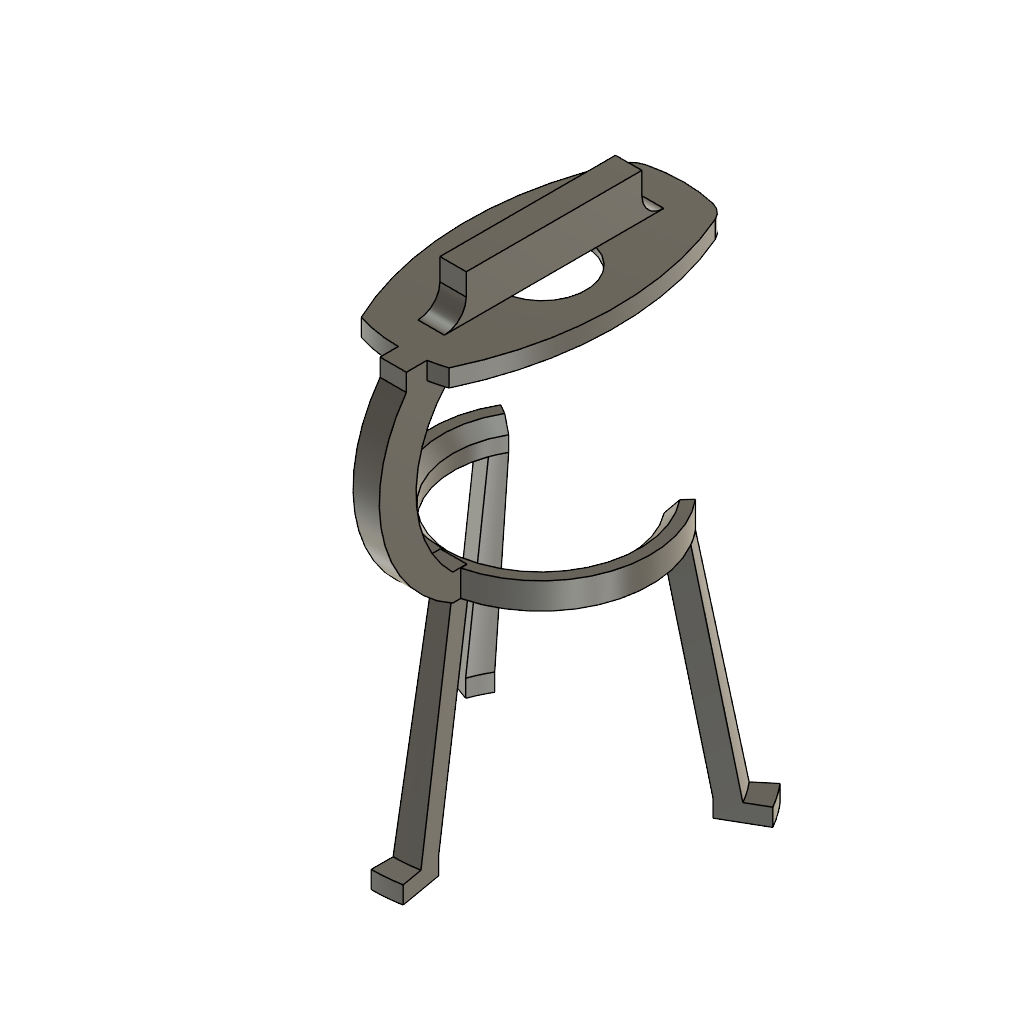
exercise 3 (Autodesk Fusion 360 design; units mm, degrees)
part number: 2026-07-30-11-30-15-373
Autodesk Fusion 360 part; units mm, degrees
note: some values were not read from the file. Set by a fixed rule: which sketch regions a step uses.
sketch "Sketch1" plane through (0, 0, 0) normal (0, 0, 1) x (1, 0, 0)
  circle A0 centre (0, 0) radius 31.75
  circle A1 centre (0, 0) radius 25.4
  dimension "d1" = 63.5
  dimension "d2" = 50.8
  constraint coincident A0.centre A1.centre
  constraint concentric A0 A1
  measures "d1" diameter of A0
  measures "d2" diameter of A1
extrude "Extrude1" add sketch "Sketch1" along normal blind 7.62 makes body 1
chamfer "Chamfer1" distance 3.175 distance2 3.175 1 edges at (-23.6811, 9.185, 7.62) measured on face at (29.4206, -2.8393, 7.62) on bodies 1
sketch "Sketch2" plane through (0, 0, 0) normal (1, 0, 0) x (0, 1, 0)
  arc A0 (-31.115, 59.4476) -> (-33.147, 7.7483) centre (-9.0465, 32.6906) ccw
  arc A1 (-46.5417, 59.4476) -> (-33.147, 0) centre (-13.9818, 35.5511) ccw
  line L0 (-33.147, 7.7483) -> (-33.147, 0)
  line L1 (-33.147, 7.7483) -> (-29.083, 7.7483)
  line L2 (-29.083, 7.7483) -> (-29.083, 0)
  line L3 (-29.083, 0) -> (-33.147, 0)
  line L4 (-33.147, 0) -> (-33.147, 7.7483)
  line L5 (-31.115, 0) -> (-31.115, 59.4476) construction
  line L6 (-46.5417, 59.4476) -> (-31.115, 59.4476)
  constraint tangent A0 A1
  constraint horizontal L1
  constraint vertical L2
  constraint horizontal L3
  constraint vertical L4
  constraint midpoint L3 L5.start
  constraint perpendicular L5 L6
extrude "Extrude2" add sketch "Sketch2" along normal blind 7.62 bodies 1
sketch "Sketch5" plane through (0, 0, 59.4476) normal (0, 0, 1) x (-1, 0, 0)
  line L0 (0, 31.115) -> (0, 46.5417)
  line L1 (0, 46.5417) -> (-7.62, 46.5417)
  line L2 (-7.62, 46.5417) -> (-7.62, 31.115)
  line L3 (-7.62, 31.115) -> (0, 31.115)
  line L4 (12.7, 39.2684) -> (-12.7, 39.2684) construction
  line L5 (-12.7, 39.2684) -> (-12.7, -39.2684) construction
  line L6 (-12.7, -39.2684) -> (12.7, -39.2684) construction
  line L7 (12.7, -39.2684) -> (12.7, 39.2684) construction
  line L8 (12.7, 39.2684) -> (-12.7, -39.2684) construction
  line L9 (-12.7, 39.2684) -> (12.7, -39.2684) construction
  arc A0 (12.7, -39.2684) -> (12.7, 39.2684) centre (-69.8788, 0) ccw
  arc A1 (12.7, 39.2684) -> (-12.7, 39.2684) centre (0, -0.0042) ccw
  arc A2 (-12.7, 39.2684) -> (-12.7, -39.2684) centre (69.8788, 0) ccw
  arc A3 (-12.7, -39.2684) -> (12.7, -39.2684) centre (0, 0.0042) ccw
  line L10 (0, 46.5417) -> (-7.62, 46.5417)
  line L11 (-7.62, 46.5417) -> (-7.62, 31.115)
  line L12 (-7.62, 31.115) -> (0, 31.115)
  line L13 (0, 31.115) -> (0, 46.5417)
  dimension "d20" = 25.4
  dimension "d21" = 78.5368
  dimension "d22" = 91.44
  dimension "d23" = 41.275
  dimension "d24" = 91.44
  dimension "d25" = 41.275
  constraint horizontal L4
  constraint perpendicular L4 L5
  constraint parallel L4 L6
  constraint parallel L5 L7
  constraint coincident L8 origin
  constraint coincident L9 origin
  constraint horizontal L10
  constraint vertical L11
  constraint horizontal L12
  constraint vertical L13
  constraint coincident L2.end L3.start
  constraint coincident L0.end L1.start
  measures "d20" distance of L5.end L6.end
  measures "d21" distance of L4.end L5.end
  measures "d22" radius of A0
  measures "d23" radius of A1
  measures "d24" radius of A2
  measures "d25" radius of A3
extrude "Extrude3" add sketch "Sketch5" along normal blind 5.08 separate body contours L0 L2 L3 A0 A1 A2 A3 L11 L12 L13 makes body 2
extrude "Extrude4" add 1 faces at (2.54, -36.2572, 59.4476) along direction (0, 0, 1) blind 5.08 on bodies 1 bodies 1 2
fillet "Fillet1" radius 6.35 1 edges at (12.7, 39.2684, 61.9876) on bodies 1
fillet "Fillet2" radius 6.35 1 edges at (-12.7, 39.2684, 61.9876) on bodies 1
sketch "Sketch6" plane through (0, 0, 64.5276) normal (0, 0, 1) x (-1, 0, 0)
  arc A0 (9.6213, -40.1338) -> (13.9635, -36.4929) centre (8.1411, -33.9587) ccw
  arc A1 (13.9635, -36.4929) -> (12.7, 39.2684) centre (-69.8788, 0) ccw
  arc A2 (12.7, 39.2684) -> (0, 41.2708) centre (0, -0.0042) ccw
  line L0 (0, 41.2708) -> (0, 46.5417)
  line L1 (0, 46.5417) -> (-7.62, 46.5417)
  line L2 (-7.62, 46.5417) -> (-7.62, 40.5613)
  arc A3 (-7.62, 40.5613) -> (-12.7, 39.2684) centre (0, -0.0042) ccw
  arc A4 (-12.7, 39.2684) -> (-13.9635, -36.4929) centre (69.8788, 0) ccw
  arc A5 (-13.9635, -36.4929) -> (-9.6213, -40.1338) centre (-8.1411, -33.9587) ccw
  arc A6 (-9.6213, -40.1338) -> (9.6213, -40.1338) centre (0, 0.0042) ccw
  circle A7 centre (-0.3341, 0.0042) radius 12.7
  dimension "d35" = 25.4
  measures "d35" diameter of A7
extrude "Extrude5" cut sketch "Sketch6" against normal blind 5.08 contours A7 bodies 1
chamfer "Chamfer2" distance 3.175 angle 45 1 edges at (12.1747, 4.5883, 59.4476) on bodies 1
sketch "Sketch7" plane through (0, 0, 64.5276) normal (0, 0, 1) x (-1, 0, 0)
  circle A0 centre (-0.3341, 0.0042) radius 12.7
  arc A1 (9.6213, -40.1338) -> (13.9635, -36.4929) centre (8.1411, -33.9587) ccw
  arc A2 (13.9635, -36.4929) -> (12.7, 39.2684) centre (-69.8788, 0) ccw
  arc A3 (12.7, 39.2684) -> (0, 41.2708) centre (0, -0.0042) ccw
  line L0 (0, 41.2708) -> (0, 46.5417)
  line L1 (0, 46.5417) -> (-7.62, 46.5417)
  line L2 (-7.62, 46.5417) -> (-7.62, 40.5613)
  arc A4 (-7.62, 40.5613) -> (-12.7, 39.2684) centre (0, -0.0042) ccw
  arc A5 (-12.7, 39.2684) -> (-13.9635, -36.4929) centre (69.8788, 0) ccw
  arc A6 (-13.9635, -36.4929) -> (-9.6213, -40.1338) centre (-8.1411, -33.9587) ccw
  arc A7 (-9.6213, -40.1338) -> (9.6213, -40.1338) centre (0, 0.0042) ccw
  line L3 (3.81, 25.4) -> (-3.81, 25.4)
  line L4 (-3.81, 25.4) -> (-3.81, -25.4)
  line L5 (-3.81, -25.4) -> (3.81, -25.4)
  line L6 (3.81, -25.4) -> (3.81, 25.4)
  line L7 (3.81, 25.4) -> (-3.81, -25.4) construction
  line L8 (-3.81, 25.4) -> (3.81, -25.4) construction
  dimension "d39" = 7.62
  dimension "d40" = 50.8
  constraint horizontal L3
  constraint perpendicular L3 L4
  constraint parallel L3 L5
  constraint parallel L4 L6
  constraint coincident L7 origin
  constraint coincident L8 origin
  measures "d39" distance of L4.end L5.end
  measures "d40" distance of L3.end L4.end
extrude "Extrude6" add sketch "Sketch7" along normal blind 12.7 contours A0 L4 L6 | A0 L3 L4 L6 | A0 L4 L5 L6 bodies 1
fillet "Fillet3" radius 6.35 1 edges at (0, -25.4, 64.5276) on bodies 1
fillet "Fillet4" radius 6.35 1 edges at (0, 25.4, 64.5276) on bodies 1
sketch "Sketch10" plane through (0, 0, 0) normal (1, 0, 0) x (0, 1, 0)
  line L0 (-31.75, 0) -> (-42.7767, -62.5353)
  line L1 (-31.75, 0) -> (31.75, 0) construction
  line L2 (-31.75, 0) -> (-25.4, 0)
  line L3 (-25.4, 0) -> (-36.4267, -62.5353)
  line L4 (-25.4, 0) -> (38.1, 0) construction
  line L5 (-36.4267, -62.5353) -> (-49.1267, -62.5353)
  line L6 (-49.1267, -62.5353) -> (-49.1267, -67.6153)
  line L7 (-49.1267, -67.6153) -> (-36.4267, -67.6153)
  line L8 (-36.4267, -67.6153) -> (-36.4267, -62.5353)
  dimension "d57" = 100
  dimension "d58" = 63.5
  dimension "d59" = 6.35
  dimension "d60" = 100
  dimension "d61" = 63.5
  dimension "d62" = 12.7
  dimension "d63" = 5.08
  constraint horizontal L1
  constraint coincident L1 L2.end
  constraint horizontal L4
  constraint horizontal L5
  constraint vertical L6
  constraint horizontal L7
  constraint vertical L8
  measures "d57" angle of L0 L1
  measures "d58" distance of L0.start L0.end
  measures "d59" distance of L0.start L2.end
  measures "d60" angle of L3 L4
  measures "d61" distance of L2.end L3.end
  measures "d62" distance of L3.end L5.end
  measures "d63" distance of L3.end L7.end
revolve "Revolve2" add sketch "Sketch10" angle 10 about axis through (0, 0, 1.75) along (0, 0, 1) bodies 1
pattern_circular "C-Pattern1" count 3 over 360 about axis through (0, 0, 1.75) along (0, 0, 1) of "Revolve2"
sketch "Sketch11" plane through (0, 0, 7.62) normal (0, 0, 1) x (-1, 0, 0)
  circle A0 centre (0, 0) radius 28.575
  line L0 (0, 31.75) -> (0, 29.083)
  line L1 (0, 29.083) -> (-7.62, 29.083)
  line L2 (-7.62, 29.083) -> (-7.62, 30.822)
  arc A1 (-7.62, 30.822) -> (0, 31.75) centre (0, 0) ccw
  line L3 (-27.4963, -15.875) -> (-37.0457, -21.3883)
  arc A2 (-37.0457, -21.3883) -> (-32.7688, -27.4963) centre (0, 0) ccw
  line L4 (-32.7688, -27.4963) -> (-24.3219, -20.4085)
  arc A3 (-27.4963, -15.875) -> (-24.3219, -20.4085) centre (0, 0) ccw
  line L5 (27.4963, -15.875) -> (37.0457, -21.3883)
  arc A4 (37.0457, -21.3883) -> (40.1969, -14.6305) centre (0, 0) ccw
  line L6 (40.1969, -14.6305) -> (29.8352, -10.8591)
  arc A5 (27.4963, -15.875) -> (29.8352, -10.8591) centre (0, 0) ccw
  line L7 (27.4963, -15.875) -> (10.16, -5.9004)
  line L8 (-24.3219, -20.4085) -> (-11.3582, -5.9004)
  line L9 (-11.3582, -5.9004) -> (10.16, -5.9004)
  line L10 (-32.7688, -27.4963) -> (0, -40.64)
  line L11 (0, -40.64) -> (37.0457, -21.3883)
  constraint coincident L5.start A5.start
  constraint coincident L4.end A3.end
  constraint horizontal L9
  constraint coincident A2.end L4.start
  constraint coincident L5.end A4.start
extrude "Extrude7" cut sketch "Sketch11" against normal blind 17.78 contours A0 L7 L8 L9 | A0 A1 L7 L8 | A1 L4 L5 L10 L11 picked at (-0.3547, -13.4585) bodies 1
